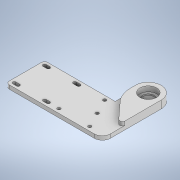
# Autodesk Inventor part: duza_czesc_pokrywka
Saved by Autodesk Inventor 2020.3 (Build 243373000, 373)
## iProperties
Created: 2021-03-12
Part Number: duza_czesc_pokrywka
Material: Generic
Document SubType Name: Modeling
Designer: patry
Density: 1 g/cm^3
Appearance: Default
Author: patry
Autodesk Inventor part; units mm, degrees
ref_plane "YZ Plane" through (0, 0, 0) normal (1, 0, 0) x (0, 1, 0)
ref_plane "XZ Plane" through (0, 0, 0) normal (0, 1, 0) x (-1, 0, 0)
ref_plane "XY Plane" through (0, 0, 0) normal (0, 0, 1) x (1, 0, 0)
sketch "Sketch1" plane through (0, 0, 0) normal (0, 1, 0) x (-1, 0, 0)
  line L0 (140, 0) -> (74, 0)
  line L1 (74, 0) -> (76, 0)
  line L2 (140, 0) -> (140, -60)
  line L3 (140, -60) -> (140, 0)
  line L4 (138, -58) -> (82, -2)
  line L5 (82, -58) -> (138, -2)
  line L6 (110, -30) -> (110, -49.4)
  line L7 (86.45, -6.45) -> (86.45, -53.55)
  line L8 (82, -58) -> (82, -2)
  line L9 (76, -58) -> (76, -2)
  line L10 (74, 0) -> (74, -60)
  line L11 (74, 0) -> (74, -60)
  circle A0 centre (86.45, -6.45) radius 2.5
  line L12 (76, -2) -> (138, -2)
  line L13 (80.45, -8.95) -> (133.55, -8.95)
  line L14 (80.45, -3.95) -> (133.55, -3.95)
  line L15 (133.55, -6.45) -> (86.45, -6.45)
  line L16 (82, -2) -> (138, -2)
  line L17 (104, -10.6) -> (110, -10.6)
  line L18 (138, -2) -> (138, -58)
  line L19 (138, -2) -> (138, -58)
  line L20 (133.55, -53.55) -> (133.55, -6.45)
  line L21 (140, -60) -> (138, -60)
  line L22 (138, -60) -> (138, -58)
  line L23 (138, -58) -> (140, -58)
  line L24 (140, -58) -> (140, -60)
  line L25 (104, -49.4) -> (110, -49.4)
  circle A1 centre (86.45, -53.55) radius 2.5
  line L26 (133.55, -51.05) -> (80.45, -51.05)
  line L27 (86.45, -53.55) -> (133.55, -53.55)
  line L28 (80.45, -56.05) -> (133.55, -56.05)
  line L29 (138, -58) -> (82, -58)
  line L30 (138, -58) -> (76, -58)
  line L31 (74, -60) -> (140, -60)
  line L32 (140, -60) -> (32, -60)
  circle A2 centre (127.55, -53.55) radius 2.5
  line L33 (104, -30) -> (104, -49.4)
  circle A3 centre (80.45, -6.45) radius 2.5
  line L34 (86.45, -53.55) -> (82, -53.55)
  line L35 (82, -58) -> (86.45, -58)
  line L36 (86.45, -58) -> (86.45, -53.55)
  line L37 (82, -53.55) -> (82, -58)
  circle A4 centre (80.45, -53.55) radius 2.5
  circle A5 centre (133.55, -53.55) radius 2.5
  line L38 (76, 0) -> (76, -2)
  line L39 (76, -2) -> (74, -2)
  line L40 (74, -2) -> (74, 0)
  line L41 (138, -2) -> (133.55, -2)
  line L42 (133.55, -2) -> (133.55, -6.45)
  line L43 (133.55, -6.45) -> (138, -6.45)
  line L44 (138, -6.45) -> (138, -2)
  circle A6 centre (127.55, -6.45) radius 2.5
  circle A7 centre (133.55, -6.45) radius 2.5
  line L45 (0, -25) -> (0, 0)
  line L46 (32, -60) -> (0, -25)
  line L47 (0, -25) -> (0, 0)
  line L48 (0, 0) -> (74, 0)
  line L49 (0, 0) -> (74, 0)
  line L50 (140, -60) -> (140, 0)
  line L51 (140, -60) -> (0, -60)
  line L52 (0, -60) -> (0, 0)
  line L53 (0, 0) -> (140, 0)
  line L54 (140, 0) -> (140, -60)
  line L55 (0, -60) -> (40, -60)
  line L56 (40, -60) -> (40, -100)
  line L57 (40, -100) -> (0, -100)
  line L58 (0, -100) -> (0, -60)
  line L59 (140, 0) -> (74, 0)
  line L60 (74, 0) -> (76, 0)
  line L61 (140, 0) -> (140, -60)
  line L62 (140, -60) -> (140, 0)
  line L63 (138, -58) -> (82, -2)
  line L64 (82, -58) -> (138, -2)
  circle A8 centre (110, -30) radius 19.4
  circle A9 centre (104, -30) radius 19.4
  line L65 (110, -30) -> (110, -49.4)
  line L66 (86.45, -6.45) -> (86.45, -53.55)
  line L67 (82, -58) -> (82, -2)
  line L68 (76, -58) -> (76, -2)
  line L69 (74, 0) -> (74, -60)
  line L70 (74, 0) -> (74, -60)
  circle A10 centre (86.45, -6.45) radius 2.5
  line L71 (76, -2) -> (138, -2)
  line L72 (80.45, -8.95) -> (133.55, -8.95)
  line L73 (80.45, -3.95) -> (133.55, -3.95)
  line L74 (133.55, -6.45) -> (86.45, -6.45)
  line L75 (82, -2) -> (138, -2)
  line L76 (104, -10.6) -> (110, -10.6)
  line L77 (138, -2) -> (138, -58)
  line L78 (138, -2) -> (138, -58)
  line L79 (133.55, -53.55) -> (133.55, -6.45)
  line L80 (140, -60) -> (138, -60)
  line L81 (138, -60) -> (138, -58)
  line L82 (138, -58) -> (140, -58)
  line L83 (140, -58) -> (140, -60)
  line L84 (104, -49.4) -> (110, -49.4)
  circle A11 centre (86.45, -53.55) radius 2.5
  line L85 (133.55, -51.05) -> (80.45, -51.05)
  line L86 (86.45, -53.55) -> (133.55, -53.55)
  line L87 (80.45, -56.05) -> (133.55, -56.05)
  line L88 (138, -58) -> (82, -58)
  line L89 (138, -58) -> (76, -58)
  line L90 (74, -60) -> (140, -60)
  line L91 (140, -60) -> (32, -60)
  circle A12 centre (127.55, -53.55) radius 2.5
  line L92 (104, -30) -> (104, -49.4)
  circle A13 centre (80.45, -6.45) radius 2.5
  line L93 (86.45, -53.55) -> (82, -53.55)
  line L94 (82, -58) -> (86.45, -58)
  line L95 (86.45, -58) -> (86.45, -53.55)
  line L96 (82, -53.55) -> (82, -58)
  circle A14 centre (80.45, -53.55) radius 2.5
  circle A15 centre (133.55, -53.55) radius 2.5
  line L97 (76, 0) -> (76, -2)
  line L98 (76, -2) -> (74, -2)
  line L99 (74, -2) -> (74, 0)
  line L100 (138, -2) -> (133.55, -2)
  line L101 (133.55, -2) -> (133.55, -6.45)
  line L102 (133.55, -6.45) -> (138, -6.45)
  line L103 (138, -6.45) -> (138, -2)
  circle A16 centre (127.55, -6.45) radius 2.5
  circle A17 centre (133.55, -6.45) radius 2.5
  line L104 (0, -25) -> (0, 0)
  line L105 (32, -60) -> (0, -25)
  line L106 (0, -25) -> (0, 0)
  line L107 (0, 0) -> (74, 0)
  line L108 (0, 0) -> (74, 0)
  line L109 (140, -60) -> (140, 0)
  line L110 (140, -60) -> (0, -60)
  line L111 (0, -60) -> (0, 0)
  line L112 (0, 0) -> (140, 0)
  line L113 (140, 0) -> (140, -60)
  line L114 (0, -60) -> (40, -60)
  line L115 (40, -60) -> (40, -100)
  line L116 (40, -100) -> (0, -100)
  line L117 (0, -100) -> (0, -60)
  line L118 (40, -100) -> (0, -60)
  line L119 (40, -60) -> (0, -100)
  circle A18 centre (104, -30) radius 10.5
  line L120 (0, -68.6498) -> (0, 0)
  line L121 (20, -80) -> (20, -180)
  line L122 (104, -30) -> (-49.3689, -120.7578)
  circle A19 centre (20, -80) radius 17
  line L123 (20, -134.4641) -> (10, -134.4641)
  line L124 (10, -134.4641) -> (10, -50)
  line L125 (10, -50) -> (20, -50)
  line L126 (20, -50) -> (20, -134.4641)
  circle A20 centre (10, -91.5992) radius 40
  circle A21 centre (10, -91.5992) radius 20
  line L127 (10, -95.8192) -> (-10, -95.8192)
  line L128 (-10, -95.8192) -> (-10, 0)
  line L129 (-10, 0) -> (10, 0)
  line L130 (10, 0) -> (10, -95.8192)
  line L131 (-10, -95.8192) -> (30, -95.8192)
  line L132 (30, -95.8192) -> (30, 0)
  line L133 (30, 0) -> (-10, 0)
  line L134 (-10, 0) -> (-10, -95.8192)
  line L135 (10, -95.8192) -> (10, -91.5992)
  line L136 (10, -91.5992) -> (9.1265, -91.5992)
  point P0 (127.55, 3.95)
  point P1 (127.55, 8.95)
  point P2 (86.45, 3.95)
  point P3 (86.45, 8.95)
  point P4 (127.55, 56.05)
  point P5 (127.55, 51.05)
  point P6 (86.45, 56.05)
  point P7 (86.45, 51.05)
  point P8 (123.7179, -16.2821)
  point P9 (131.05, -8.95)
  point P10 (88.95, -8.95)
  point P11 (88.2178, -8.2178)
  point P12 (86.45, -8.95)
  point P13 (82, -3.95)
  point P14 (135.3178, -55.3178)
  point P15 (127.55, -56.05)
  point P16 (127.55, -51.05)
  point P17 (131.05, -51.05)
  point P18 (123.7179, -43.7179)
  point P19 (86.45, -51.05)
  point P20 (86.45, -56.05)
  point P21 (86.45, -3.95)
  point P22 (127.55, -8.95)
  point P23 (127.55, -3.95)
  point P24 (86.45, -8.95)
  point P25 (86.45, -3.95)
  point P26 (127.55, -56.05)
  point P27 (127.55, -51.05)
  point P28 (127.55, -8.95)
  point P29 (127.55, -3.95)
  point P30 (86.45, -51.05)
  point P31 (86.45, -56.05)
  point P32 (127.55, 3.95)
  point P33 (127.55, 8.95)
  point P34 (86.45, 3.95)
  point P35 (86.45, 8.95)
  point P36 (127.55, 56.05)
  point P37 (127.55, 51.05)
  point P38 (86.45, 56.05)
  point P39 (86.45, 51.05)
  point P40 (123.7179, -16.2821)
  point P41 (131.05, -8.95)
  point P42 (88.95, -8.95)
  point P43 (88.2178, -8.2178)
  point P44 (86.45, -8.95)
  point P45 (82, -3.95)
  point P46 (135.3178, -55.3178)
  point P47 (127.55, -56.05)
  point P48 (127.55, -51.05)
  point P49 (131.05, -51.05)
  point P50 (123.7179, -43.7179)
  point P51 (86.45, -51.05)
  point P52 (86.45, -56.05)
  point P53 (86.45, -3.95)
  point P54 (127.55, -8.95)
  point P55 (127.55, -3.95)
  point P56 (30, -60)
  point P57 (88.95, -51.05)
  point P58 (88.2178, -51.7822)
  point P59 (88.2178, -8.2178)
  point P60 (88.95, -8.95)
  point P61 (-10, -91.5992)
  point P62 (30, -91.5992)
  point P63 (30, -60)
  point P64 (104.0094, -10.6)
  point P65 (109.9957, -10.6)
  dimension "d0" = 40
  dimension "d1" = 40
  dimension "d43" = 40
  dimension "d44" = 40
  dimension "d45" = 21
  dimension "d46" = 100
  dimension "d47" = 34
  dimension "d48" = 10
  dimension "d49" = 80
  dimension "d50" = 40
  dimension "d51" = 20
  dimension "d81" = 4.22
  constraints: 274 end point, 22 centre point, 20 point on circle, 16 equal length, 15 point on line, 11 perpendicular, 9 horizontal, 5 coincident, 1 midpoint, 1 vertical
  measures "d0" distance of L56.end L57.end
  measures "d1" distance of L55.end L56.end
  measures "d43" distance of L115.end L116.end
  measures "d44" distance of L114.end L115.end
  measures "d45" diameter of A18
  measures "d46" distance of L121.start L121.end
  measures "d47" diameter of A19
  measures "d48" distance of L124.end L125.end
  measures "d49" diameter of A20
  measures "d50" diameter of A21
  measures "d51" distance of L128.end L129.end
  measures "d81" distance of L135.start L135.end
extrude "Extrusion5" add sketch "Sketch1" along normal blind 6 contours L2 L23 L18 L12 L38 L0 | L38 L39 L10 L0 | L2 L21 L22 L23 | L10 L122 L32 A20 L132 L48 | L12 L8 L14 A3 L13 L122 L9 | L9 L122 L10 L39 | L29 L36 L28 A5 L4 | L4 A5 L20 A7 L43 L18 | L22 L31 L10 L122 L9 L30 L29 | L132 A20 L46 L130 L48 | L122 L8 L26 A4 L28 L30 L9 | L12 L42 L14 L4 | L4 L14 L8 | L43 A7 L5 L18 | L29 L5 L28 L36 | L10 L32 L122 | L130 L46 L45 L48 | L132 L46 A20 | A20 L32 L46 L132 | L122 L7 L26 L8 | L8 L13 L7 A9 L122 | L12 L5 A7 L42 | L8 L28 L5 | A1 L27 A2 L28 | L45 L52 A20 L128 L129 | L130 L124 A20 L52 L46 | L46 A20 L126 L125 L130 | L46 L132 L51 L126 A20 | L46 L51 L132 | L122 A9 L5 L26 L7 | L7 A9 L122 | L14 A6 L15 A0 | L26 L4 A8 L5 L13 L20 | A1 L5 L26 A2 L27 | L125 L126 A20 L124 | L126 L51 L124 A20 | L132 A19 L126 L51 | L26 L5 A1 | L13 L4 A9 L7 | A0 L4 L13 | A9 L7 | L7 A9 L4 A8 L122 | L122 A8 L5 A9 | L15 A6 L13 L4 A0 | L26 L5 A9 L25 A8 L4 | L5 A8 L17 A9 L4 L13 | A20 L124 L51 L52 | L52 L58 A21 L128 A20 | L126 A19 L124 L51 | L132 L119 A21 L126 A19 | L5 A8 L33 A9 | L122 A18 L5 A8 | A8 L4 A18 L122 | A8 L6 A9 L4 | L4 A9 L5 A8 | L5 A9 A8 | L118 A19 A21 L58 | L51 L124 A19 L118 | A21 L58 L122 L127 | L132 L122 A21 L119 | L126 A21 L118 L124 A19 | A9 A8 L4 | L5 A18 L33 A8 | A9 A8 L25 | L33 A8 A9 | A8 A9 L5 A18 L4 | L122 L33 L5 A18 | A18 L4 L5 L33 L122 | A9 L6 A18 L4 | L4 A18 L5 A9 | A8 A9 L6 | A8 A9 L17 | A21 L121 L57 | L57 L121 A19 L131 A21 | L132 L118 A21 L122 | A21 L124 L57 L121 | A19 L124 L118 | L118 L124 A21 A19 | A21 L127 L122 | L122 L127 L58 L57 L124 A21 | A21 A19 L122 L58 | A21 L122 L119 | L119 L122 L126 A21 | L126 L122 L118 A21 | L5 L33 A18 | L33 A18 L6 A9 A8 | A18 L5 L4 | A18 L6 L4 | L4 L5 A18 | L57 L124 L131 A19 L121 | L131 A19 A21 | L132 A21 L118 | A21 L118 L119 L122 | L118 A21 L124 | A21 L124 L122 A19 | L122 L58 L127 | L122 A19 L119 L127 L58 | L119 L126 L122 | L126 L118 L122 | L118 L122 L124 A21 | L5 L6 A18 L33 | L57 L119 L127 L124 | A19 L131 L121 | L121 L131 A19 | A19 L131 L121 L118 A21 | L122 L124 L119 A19 | L127 L119 L58 | L119 L124 L122 L118 | L121 L131 A19 L124 L119 | L127 L119 A19 L124 | L124 A19 L131 | L119 L124 A19
sketch "Sketch7" plane through (0, 6, 0) normal (0, 1, 0) x (1, 0, 0)
  line L0 (0, 0) -> (-140, 0)
  line L1 (-32, 0) -> (0, 0)
  line L2 (-140, 0) -> (-140, 60)
  line L3 (-140, 60) -> (-32, 60)
  line L4 (0, 25) -> (0, 0)
  line L5 (0, 0) -> (0, 25)
  line L6 (0, 0) -> (0, 25)
  line L7 (0, 25) -> (-32, 60)
  line L8 (-32, 60) -> (10, 14.0625)
  line L9 (10, 0) -> (10, 91.5992) projected
  arc A0 (10, 91.5992) -> (-30, 91.5992) centre (-10, 91.5992) ccw projected
  circle A1 centre (-10, 91.5992) radius 20
  line L10 (-30, 91.5992) -> (-30, 60) projected
  line L11 (-30, 91.5992) -> (-30, 60)
  line L12 (-30, 60) -> (-32, 60)
  line L13 (10, 91.5992) -> (10, 14.0625)
  line L14 (0, 25) -> (0, 0)
  line L15 (135, 0) -> (-10, 0)
  line L16 (-10, 0) -> (0, 0)
  line L17 (0, 0) -> (0, 25)
  line L18 (10, 25) -> (10, 0)
  line L19 (-32, 60) -> (-22, 60)
  line L20 (-22, 60) -> (10, 25)
  line L21 (-69, 60) -> (-32, 60)
  line L22 (0, 25) -> (-32, 60)
  point P0 (6.0531, 31.6206)
  constraints: 42 end point, 3 vertical, 2 point on line, 1 coincident, 1 collinear, 1 horizontal, 1 horizontal alignment, 1 perpendicular, 2 other
fillet "Fillet10" radius 5 2 edges at (-140, 3, -60) (-140, 3, 0)
fillet "Fillet11" radius 12.5 1 edges at (10, 3, 0)
sketch "Sketch10" plane through (0, 0, 0) normal (0, -1, 0) x (1, 0, 0)
  line L0 (74, 60) -> (0, 60)
  line L1 (0, 60) -> (0, 0)
  line L2 (0, 0) -> (74, 0)
  line L3 (74, 0) -> (74, 60)
  arc A0 (80.45, 8.95) -> (80.45, 3.95) centre (80.45, 6.45) ccw
  line L4 (80.45, 6.45) -> (0, 6.45)
  arc A1 (80.45, 56.05) -> (80.45, 51.05) centre (80.45, 53.55) ccw
  line L5 (80.45, 53.55) -> (0, 53.55)
  line L6 (0, 20) -> (0, 80)
  line L7 (74, 18.2674) -> (74, 55)
  line L8 (74, 53.55) -> (64, 53.55)
  line L9 (64, 53.55) -> (64, 6.45)
  line L10 (64, 53.55) -> (40, 53.55)
  line L11 (64, 6.45) -> (40, 6.45)
  line L12 (40, 6.45) -> (16, 6.45)
  line L13 (16, 6.45) -> (40, 53.55)
  line L14 (40, 53.55) -> (28.6497, 31.2751)
  arc A2 (104, 49.4) -> (98.7489, 11.3242) centre (104, 30) ccw
  line L15 (104, 30) -> (28, 30)
  line L16 (-53.55, 64) -> (-53.55, 40)
  line L17 (-18.2674, 74) -> (-55, 74)
  line L18 (-30, 104) -> (-30, 28)
  line L19 (-53.55, 40) -> (-31.2751, 28.6497)
  line L20 (-53.55, 64) -> (-6.45, 64)
  line L21 (0, 74) -> (-60, 74)
  line L22 (-6.45, 64) -> (-6.45, 40)
  line L23 (-60, 74) -> (-60, 0)
  line L24 (-53.55, 80.45) -> (-53.55, 0)
  line L25 (-6.45, 80.45) -> (-6.45, 0)
  line L26 (0, 0) -> (0, 74)
  line L27 (-6.45, 40) -> (-6.45, 16)
  line L28 (-6.45, 16) -> (-53.55, 40)
  line L29 (-60, 0) -> (0, 0)
  arc A3 (-56.05, 80.45) -> (-51.05, 80.45) centre (-53.55, 80.45) ccw
  line L30 (-53.55, 74) -> (-53.55, 64)
  arc A4 (-8.95, 80.45) -> (-3.95, 80.45) centre (-6.45, 80.45) ccw
  line L31 (-20, 0) -> (-80, 0)
  arc A5 (-49.4, 104) -> (-11.3242, 98.7489) centre (-30, 104) ccw
  line L32 (-64, -53.55) -> (-40, -53.55)
  line L33 (-74, -18.2674) -> (-74, -55)
  line L34 (-104, -30) -> (-28, -30)
  line L35 (-40, -53.55) -> (-28.6497, -31.2751)
  line L36 (-64, -53.55) -> (-64, -6.45)
  line L37 (-74, 0) -> (-74, -60)
  line L38 (-64, -6.45) -> (-40, -6.45)
  line L39 (-74, -60) -> (0, -60)
  line L40 (-80.45, -53.55) -> (0, -53.55)
  line L41 (-80.45, -6.45) -> (0, -6.45)
  line L42 (0, 0) -> (-74, 0)
  line L43 (-40, -6.45) -> (-16, -6.45)
  line L44 (-16, -6.45) -> (-40, -53.55)
  line L45 (0, -60) -> (0, 0)
  arc A6 (-80.45, -56.05) -> (-80.45, -51.05) centre (-80.45, -53.55) ccw
  line L46 (-74, -53.55) -> (-64, -53.55)
  arc A7 (-80.45, -8.95) -> (-80.45, -3.95) centre (-80.45, -6.45) ccw
  line L47 (0, -20) -> (0, -80)
  arc A8 (-104, -49.4) -> (-98.7489, -11.3242) centre (-104, -30) ccw
  line L48 (53.55, -64) -> (53.55, -40)
  line L49 (18.2674, -74) -> (55, -74)
  line L50 (30, -104) -> (30, -28)
  line L51 (53.55, -40) -> (31.2751, -28.6497)
  line L52 (53.55, -64) -> (6.45, -64)
  line L53 (0, -74) -> (60, -74)
  line L54 (6.45, -64) -> (6.45, -40)
  line L55 (60, -74) -> (60, 0)
  line L56 (53.55, -80.45) -> (53.55, 0)
  line L57 (6.45, -80.45) -> (6.45, 0)
  line L58 (0, 0) -> (0, -74)
  line L59 (6.45, -40) -> (6.45, -16)
  line L60 (6.45, -16) -> (53.55, -40)
  line L61 (60, 0) -> (0, 0)
  arc A9 (56.05, -80.45) -> (51.05, -80.45) centre (53.55, -80.45) ccw
  line L62 (53.55, -74) -> (53.55, -64)
  arc A10 (8.95, -80.45) -> (3.95, -80.45) centre (6.45, -80.45) ccw
  line L63 (20, 0) -> (80, 0)
  arc A11 (49.4, -104) -> (11.3242, -98.7489) centre (30, -104) ccw
  dimension "d66" = 10
  dimension "d67" = 24
  dimension "d68" = 24
  dimension "d69" = 24
  dimension "d72" = 360
  constraints: 128 end point, 40 point on line, 24 point on circle, 12 centre point, 3 parallel, 3 perpendicular, 2 coincident, 1 horizontal, 1 midpoint, 187 other
  measures "d66" distance of L8.start L8.end
  measures "d67" distance of L8.end L10.end
  measures "d68" distance of L9.end L11.end
  measures "d69" distance of L11.end L12.end
hole "Hole3" at (-40, 0, -53.55) at (-28, 0, -30) at (-16, 0, -6.45) at (-64, 0, -6.45) direction (0, 1, 0) diameter 5 end through all
extrude "Extrusion9" add sketch "Sketch7" along normal blind 6 contours L10 A1 L9 L20 L19 | A0 A1
sketch "Sketch11" plane through (0, 12, 0) normal (0, 1, 0) x (1, 0, 0)
  arc A0 (10, 91.5992) -> (-30, 91.5992) centre (-10, 91.5992) ccw projected
  circle A1 centre (-10, 91.5992) radius 13
  point P0 (0, 0)
  dimension "d89" = 26
  constraints: 1 centre point, 1 coincident
  measures "d89" diameter of A1
extrude "Extrusion12" cut sketch "Sketch11" against normal blind 8
sketch "Sketch12" plane through (-10, 4, -91.5992) normal (0, 1, 0) x (1, 0, 0)
  circle A0 centre (0, 0) radius 9
  point P0 (10, -91.5992)
  dimension "d92" = 18
  constraints: 1 centre point
  measures "d92" diameter of A0
extrude "Extrusion13" cut sketch "Sketch12" against normal blind 2
fillet "Fillet13" radius 4 1 edges at (10, 9, -25)
fillet "Fillet14" radius 40 1 edges at (-30, 9, -60)
body "Solid1"
